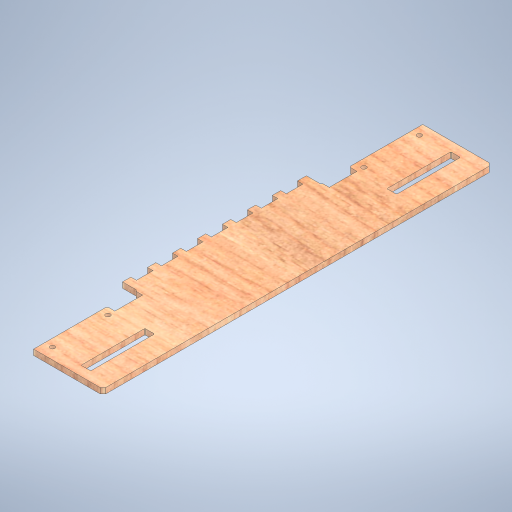
# Autodesk Inventor part: фанера_жлектроника_новая
Saved by Autodesk Inventor 2023.1 (Build 271208000, 208)
## iProperties
Created: 2026-02-21
Part Number: фанера_жлектроника_новая
Material: Типовые
Document SubType Name: Modeling
Designer: DELL
Density: 1 g/cm^3
Appearance: Береза — натуральный — полированный
Author: DELL
Autodesk Inventor part; units mm, degrees
ref_plane "YZ Plane" through (0, 0, 0) normal (1, 0, 0) x (0, 1, 0)
ref_plane "XZ Plane" through (0, 0, 0) normal (0, 1, 0) x (-1, 0, 0)
ref_plane "XY Plane" through (0, 0, 0) normal (0, 0, 1) x (1, 0, 0)
sketch "Эскиз1" plane through (0, 0, 0) normal (0, 1, 0) x (-1, 0, 0)
  line L0 (-25, -140.25) -> (25, -140.25)
  line L1 (25, -140.25) -> (25, 140.25)
  line L2 (25, 140.25) -> (-25, 140.25)
  line L3 (-25, 140.25) -> (-25, -140.25)
  line L4 (-25, -140.25) -> (25, 140.25) construction
  line L5 (25, -140.25) -> (-25, 140.25) construction
  circle A0 centre (19.4, 132.25) radius 1.65
  circle A1 centre (19.4, 92.25) radius 1.65
  line L6 (-25, 0) -> (0, 0)
  line L7 (25, 87.25) -> (19.4, 87.25)
  line L8 (19.4, 87.25) -> (19.4, 67.25)
  line L9 (19.4, 67.25) -> (25, 67.25)
  line L10 (25, 67.25) -> (25, 87.25)
  line L11 (-9.2, 133.25) -> (-2.2, 133.25)
  line L12 (-2.2, 133.25) -> (-2.2, 87.25)
  line L13 (-2.2, 87.25) -> (-9.2, 87.25)
  line L14 (-9.2, 87.25) -> (-9.2, 133.25)
  circle A2 centre (19.4, -132.25) radius 1.65
  circle A3 centre (19.4, -92.25) radius 1.65
  line L15 (25, -87.25) -> (19.4, -87.25)
  line L16 (19.4, -87.25) -> (19.4, -67.25)
  line L17 (19.4, -67.25) -> (25, -67.25)
  line L18 (-9.2, -133.25) -> (-2.2, -133.25)
  line L19 (-2.2, -133.25) -> (-2.2, -87.25)
  line L20 (-2.2, -87.25) -> (-9.2, -87.25)
  line L21 (-9.2, -87.25) -> (-9.2, -133.25)
  point P0 (25, -87.25)
  point P1 (25, -67.25)
  dimension "d0" = 50
  dimension "d1" = 280.5
  dimension "d2" = 3.3
  dimension "d3" = 3.3
  dimension "d4" = 5.6
  dimension "d5" = 5.6
  dimension "d6" = 8
  dimension "d7" = 40
  dimension "d8" = 20
  dimension "d9" = 5
  dimension "d10" = 5.6
  dimension "d11" = 7
  dimension "d12" = 46
  dimension "d13" = 7
  dimension "d17" = 28.6
  constraints: 44 end point, 10 symmetric about line, 6 parallel, 4 centre point, 4 horizontal, 3 midpoint, 3 perpendicular, 1 point on line, 2 other
  measures "d0" distance of L2.end L1.end
  measures "d1" distance of L1.end L0.end
  measures "d2" diameter of A0
  measures "d3" diameter of A1
  measures "d4" distance from line of L1 A0.centre
  measures "d5" distance from line of L1 A1.centre
  measures "d6" distance from line of L2 A0.centre
  measures "d7" distance of A1.centre A0.centre
  measures "d8" distance of L7.end L8.end
  measures "d9" distance from line of L7 A1.centre
  measures "d10" distance of L8.end L9.end
  measures "d11" distance of L12.end L13.end
  measures "d12" distance of L11.end L12.end
  measures "d13" distance between parallel lines of L2 L11
  measures "d17" distance from line of L14 A1.centre
extrude "Выдавливание1" add sketch "Эскиз1" along normal blind 4 contours L3 L2 L1 L7 L8 L9 L17 L16 L15 L0
chamfer "Фаска1" distance 2 angle 45 2 edges at (25, 2, -140.25) (25, 2, 140.25)
chamfer "Фаска2" distance 0.5 angle 45 8 edges at (9.2, 2, 87.25) (2.2, 2, 87.25) (9.2, 2, 133.25) (2.2, 2, 133.25) (2.2, 2, -87.25) (2.2, 2, -133.25) (9.2, 2, -133.25) (9.2, 2, -87.25)
chamfer "Фаска3" distance 1 angle 45 4 edges at (-25, 2, -87.25) (-25, 2, -67.25) (-25, 2, 87.25) (-25, 2, 67.25)
sketch "Эскиз2" plane through (0, 0, 0) normal (0, -1, 0) x (1, 0, 0)
  line L0 (-25, -66.25) -> (-25, 66.25) projected
  line L1 (-25, -66.25) -> (-34.9, -66.25)
  line L2 (-34.9, -66.25) -> (-34.9, 66.25)
  line L3 (-34.9, 66.25) -> (-25, 66.25)
  line L4 (-25, 66.25) -> (-25, -66.25)
  point P0 (0, 0)
  dimension "d27" = 9.9
  constraints: 8 end point, 2 parallel, 1 horizontal, 1 perpendicular
  measures "d27" distance of L2.end L3.end
extrude "Выдавливание2" add sketch "Эскиз2" against normal blind 4
sketch "Эскиз3" plane through (0, 4, 0) normal (0, 1, 0) x (1, 0, 0)
  line L0 (-34.9, -66.25) -> (-34.9, 66.25) projected
  line L1 (-34.9, -60.25) -> (-30.9, -60.25)
  line L2 (-30.9, -60.25) -> (-30.9, -48.25)
  line L3 (-30.9, -48.25) -> (-34.9, -48.25)
  line L4 (-34.9, -48.25) -> (-34.9, -60.25)
  line L5 (-34.9, -66.25) -> (-25, -66.25) projected
  line L6 (-34.9, -42.25) -> (-30.9, -42.25)
  line L7 (-30.9, -42.25) -> (-30.9, -30.25)
  line L8 (-30.9, -30.25) -> (-34.9, -30.25)
  line L9 (-34.9, -30.25) -> (-34.9, -42.25)
  line L10 (-34.9, -24.25) -> (-30.9, -24.25)
  line L11 (-30.9, -24.25) -> (-30.9, -12.25)
  line L12 (-30.9, -12.25) -> (-34.9, -12.25)
  line L13 (-34.9, -12.25) -> (-34.9, -24.25)
  line L14 (-34.9, -6.25) -> (-30.9, -6.25)
  line L15 (-30.9, -6.25) -> (-30.9, 5.75)
  line L16 (-30.9, 5.75) -> (-34.9, 5.75)
  line L17 (-34.9, 5.75) -> (-34.9, -6.25)
  line L18 (-34.9, 11.75) -> (-30.9, 11.75)
  line L19 (-30.9, 11.75) -> (-30.9, 23.75)
  line L20 (-30.9, 23.75) -> (-34.9, 23.75)
  line L21 (-34.9, 23.75) -> (-34.9, 11.75)
  line L22 (-34.9, 29.75) -> (-30.9, 29.75)
  line L23 (-30.9, 29.75) -> (-30.9, 41.75)
  line L24 (-30.9, 41.75) -> (-34.9, 41.75)
  line L25 (-34.9, 41.75) -> (-34.9, 29.75)
  line L26 (-34.9, 47.75) -> (-30.9, 47.75)
  line L27 (-30.9, 47.75) -> (-30.9, 59.75)
  line L28 (-30.9, 59.75) -> (-34.9, 59.75)
  line L29 (-34.9, 59.75) -> (-34.9, 47.75)
  point P0 (0, 0)
  point P1 (-32.9, -60.25)
  point P2 (-32.9, -42.25)
  point P3 (-32.9, -24.25)
  point P4 (-32.9, -6.25)
  point P5 (-32.9, 11.75)
  point P6 (-32.9, 29.75)
  point P7 (-32.9, 47.75)
  dimension "d32" = 4
  dimension "d33" = 12
  dimension "d34" = 6
  dimension "d37" = 18
  constraints: 56 end point, 2 parallel, 1 horizontal, 1 midpoint, 1 perpendicular, 1 point on line, 1 vertical, 54 other
  measures "d32" distance of L3.end L2.end
  measures "d33" distance of L2.end L1.end
  measures "d34" distance from line of L5 point (-32.9, -60.25)
  measures "d37" distance of L2.end L7.end
extrude "Выдавливание3" cut sketch "Эскиз3" against normal blind 4
